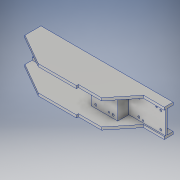
# Autodesk Inventor part: xtion_heatsink_mod
Saved by Autodesk Inventor 2017 (Build 210142000, 142)
## iProperties
Created: 2016-11-14
Part Number: xtion_heatsink_mod
Material: Aluminum 6061
Document SubType Name: Modeling
Designer: Alistair
Density: 2.7 g/cm^3
Appearance: Aluminum - Flat
Author: Alistair
Autodesk Inventor part; units mm, degrees
ref_plane "YZ Plane" through (0, 0, 0) normal (1, 0, 0) x (0, 1, 0)
ref_plane "XZ Plane" through (0, 0, 0) normal (0, 1, 0) x (-1, 0, 0)
ref_plane "XY Plane" through (0, 0, 0) normal (0, 0, 1) x (1, 0, 0)
sketch "Sketch1" plane through (0, 0, 0) normal (0, 0, 1) x (1, 0, 0)
  line L0 (-75, -10.5) -> (75, -10.5)
  line L1 (82, -9.5) -> (82, 9.5)
  line L2 (75, 10.5) -> (-75, 10.5)
  line L3 (-82, 9.5) -> (-82, -9.5)
  line L4 (-82, -10.5) -> (82, 10.5) construction
  line L5 (82, -10.5) -> (-82, 10.5) construction
  line L6 (75, 10.5) -> (82, 9.5)
  line L7 (0, 0) -> (27.9529, 0)
  line L8 (0, 0) -> (0, 6.9962)
  line L9 (-75, 10.5) -> (-82, 9.5)
  line L10 (75, -10.5) -> (82, -9.5)
  line L11 (-75, -10.5) -> (-82, -9.5)
  dimension "d0" = 21
  dimension "d1" = 164
  dimension "d4" = 7
  dimension "d5" = 1
  constraints: 24 end point, 6 symmetric about line, 5 point on line, 2 horizontal, 2 midpoint, 2 parallel, 1 perpendicular, 1 vertical
  measures "d0" distance of L5.end L4.start
  measures "d1" distance of L4.end L5.end
  measures "d4" distance from line of L1 L2.start
  measures "d5" vertical distance of L1.end L2.start
extrude "Extrusion1" add sketch "Sketch1" along normal blind 29
sketch "Sketch2" plane through (0, 0, 29) normal (0, 0, 1) x (1, 0, 0)
  line L0 (75, 10.5) -> (-75, 10.5) projected
  line L1 (-75, 10.5) -> (-82, 9.5) projected
  line L2 (-82, 9.5) -> (-82, -9.5) projected
  line L3 (-82, -9.5) -> (-75, -10.5) projected
  line L4 (-75, -10.5) -> (75, -10.5) projected
  line L5 (75, -10.5) -> (82, -9.5) projected
  line L6 (82, -9.5) -> (82, 9.5) projected
  line L7 (82, 9.5) -> (75, 10.5) projected
  line L8 (-74.8579, 8.5) -> (74.8579, 8.5)
  line L9 (74.8579, 8.5) -> (82, 7.4797)
  line L10 (82, -7.4797) -> (74.8579, -8.5)
  line L11 (74.8579, -8.5) -> (-74.8579, -8.5)
  line L12 (-74.8579, -8.5) -> (-82, -7.4797)
  line L13 (-82, 7.4797) -> (-74.8579, 8.5)
  point P0 (0, 0)
  dimension "d6" = 2
  constraints: 12 end point, 4 point on line
  measures "d6" distance between parallel lines of L0 L8
extrude "Extrusion2" cut sketch "Sketch2" against normal blind 15 contours L6 L10 L11 L12 L2 L13 L8 L9
sketch "Sketch3" plane through (0, 0, 14) normal (0, 0, 1) x (1, 0, 0)
  line L0 (-82, 7.4797) -> (-74.8579, 8.5) projected
  line L1 (-74.8579, 8.5) -> (74.8579, 8.5) projected
  line L2 (-74.8579, -8.5) -> (-82, -7.4797) projected
  line L3 (74.8579, -8.5) -> (-74.8579, -8.5) projected
  line L4 (82, -7.4797) -> (74.8579, -8.5) projected
  line L5 (74.8579, 8.5) -> (82, 7.4797) projected
  arc A0 (-82, -4.5) -> (-82, 4.5) centre (-83.875, 0) ccw
  line L6 (0, 0) -> (-13.589, 0)
  line L7 (-82, -7.4797) -> (-82, -4.5)
  line L8 (-82, 4.5) -> (-82, 7.4797)
  line L9 (0, 0) -> (0, 3.5906)
  arc A1 (82, 4.5) -> (82, -4.5) centre (83.875, 0) ccw
  line L10 (82, 7.4797) -> (82, 4.5)
  line L11 (82, -4.5) -> (82, -7.4797)
  arc A2 (-80.5, -5.4083) -> (-80.5, 5.4083) centre (-83.875, 0) ccw
  line L12 (-80.5, -5.4083) -> (-80.5, -7.694)
  line L13 (80.5, -7.694) -> (80.5, -5.4083)
  arc A3 (80.5, 5.4083) -> (80.5, -5.4083) centre (83.875, 0) ccw
  line L14 (80.5, 5.4083) -> (80.5, 7.694)
  line L15 (-80.5, 7.694) -> (-80.5, 5.4083)
  line L16 (-74.8579, 8.5) -> (74.8579, 8.5) projected
  line L17 (74.8579, -8.5) -> (-74.8579, -8.5) projected
  line L18 (10.5, 8.5) -> (30.5, 8.5)
  line L19 (30.5, 8.5) -> (30.5, -8.5)
  line L20 (30.5, -8.5) -> (10.5, -8.5)
  line L21 (10.5, -8.5) -> (10.5, 8.5)
  line L22 (82, -4.5) -> (82, 4.5)
  line L23 (82, -9.5) -> (82, 9.5) projected
  line L24 (-82, 4.5) -> (-82, -4.5)
  dimension "d10" = 9
  dimension "d11" = 3
  dimension "d12" = 1.5
  dimension "d13" = 1.5
  dimension "d14" = 1.5
  dimension "d15" = 1.5
  dimension "d16" = 1.5
  dimension "d17" = 1.5
  dimension "d18" = 20
  dimension "d19" = 51.5
  constraints: 32 end point, 10 point on circle, 9 point on line, 4 centre point, 4 parallel, 3 symmetric about line, 3 vertical, 2 horizontal, 1 collinear, 1 perpendicular, 1 other
  measures "d10" distance of L7.end L8.start
  measures "d11" distance edge to line of A0 L7
  measures "d12" radial gap between concentric circles of A0 A2
  measures "d13" radial gap between concentric circles of A1 A3
  measures "d14" distance between parallel lines of L10 L14
  measures "d15" distance between parallel lines of L11 L13
  measures "d16" distance between parallel lines of L8 L15
  measures "d17" distance between parallel lines of L7 L12
  measures "d18" distance between parallel lines of L19 L21
  measures "d19" distance between parallel lines of L11 L19
extrude "Extrusion3" cut sketch "Sketch3" against normal blind 7.5 contours L0 L1 L21 L3 L2 L12 A2 L15 | L1 L5 L14 A3 L13 L4 L3 L19 | L22 A1
sketch "Sketch4" plane through (0, 0, 6.5) normal (0, 0, 1) x (1, 0, 0)
  line L0 (-82, -4.5) -> (-82, 4.5) projected
  arc A0 (-82, -4.5) -> (-82, 4.5) centre (-83.875, 0) ccw projected
  line L1 (82, 4.5) -> (82, -4.5) projected
  arc A1 (82, 4.5) -> (82, -4.5) centre (83.875, 0) ccw projected
  line L2 (30.5, -8.5) -> (30.5, 8.5) projected
  line L3 (74.8579, -8.5) -> (30.5, -8.5) projected
  line L4 (80.5, -7.694) -> (74.8579, -8.5) projected
  line L5 (80.5, -5.4083) -> (80.5, -7.694) projected
  arc A2 (80.5, 5.4083) -> (80.5, -5.4083) centre (83.875, 0) ccw projected
  line L6 (80.5, 7.694) -> (80.5, 5.4083) projected
  line L7 (74.8579, 8.5) -> (80.5, 7.694) projected
  line L8 (30.5, 8.5) -> (74.8579, 8.5) projected
  line L9 (10.5, -8.5) -> (10.5, 8.5) projected
  line L10 (-74.8579, 8.5) -> (10.5, 8.5) projected
  line L11 (-80.5, 7.694) -> (-74.8579, 8.5) projected
  line L12 (-80.5, 5.4083) -> (-80.5, 7.694) projected
  arc A3 (-80.5, -5.4083) -> (-80.5, 5.4083) centre (-83.875, 0) ccw projected
  line L13 (-80.5, -7.694) -> (-80.5, -5.4083) projected
  line L14 (-74.8579, -8.5) -> (-80.5, -7.694) projected
  line L15 (10.5, -8.5) -> (-74.8579, -8.5) projected
  line L16 (4, 8.5) -> (4, -8.5)
  line L17 (-74.8579, 8.5) -> (74.8579, 8.5) projected
  line L18 (74.5, 8.5) -> (74.5, -8.5)
  line L19 (74.8579, -8.5) -> (-74.8579, -8.5) projected
  line L20 (63.5, 8.5) -> (63.5, -8.5)
  line L21 (-58, 6.5) -> (-35.889, 6.5)
  line L22 (-35.889, 6.5) -> (-35.889, -6.5)
  line L23 (-35.889, -6.5) -> (-58, -6.5)
  line L24 (-58, -6.5) -> (-58, 6.5)
  point P0 (0, 0)
  dimension "d22" = 6.5
  dimension "d23" = 7.5
  dimension "d24" = 11
  dimension "d25" = 24
  dimension "d26" = 2
  dimension "d27" = 2
  dimension "d28" = 22.111
  constraints: 14 end point, 6 point on line, 4 perpendicular, 2 parallel, 1 horizontal
  measures "d22" distance between parallel lines of L9 L16
  measures "d23" distance between parallel lines of L1 L18
  measures "d24" distance between parallel lines of L18 L20
  measures "d25" distance between parallel lines of L24 L0
  measures "d26" distance between parallel lines of L17 L21
  measures "d27" distance between parallel lines of L15 L23
  measures "d28" distance between parallel lines of L24 L22
extrude "Extrusion4" cut sketch "Sketch4" against normal through all contours L0 A0 | L1 A1 | L20 L8 L18 L3 | L15 L16 L10 L9 | L21 L22 L23 L24
sketch "Sketch5" plane through (0, 0, 0) normal (0, 0, -1) x (-1, 0, 0)
  line L0 (-4, -8.5) -> (-4, 8.5) projected
  line L1 (74.8579, 8.5) -> (-4, 8.5) projected
  line L2 (80.5, 7.694) -> (74.8579, 8.5) projected
  line L3 (80.5, 5.4083) -> (80.5, 7.694) projected
  arc A0 (80.5, 5.4083) -> (80.5, -5.4083) centre (83.875, 0) ccw projected
  line L4 (80.5, -7.694) -> (80.5, -5.4083) projected
  line L5 (74.8579, -8.5) -> (80.5, -7.694) projected
  line L6 (-4, -8.5) -> (74.8579, -8.5) projected
  line L7 (58, -6.5) -> (58, 6.5) projected
  line L8 (58, 6.5) -> (35.889, 6.5) projected
  line L9 (35.889, 6.5) -> (35.889, -6.5) projected
  line L10 (35.889, -6.5) -> (58, -6.5) projected
  line L11 (-63.5, -8.5) -> (-63.5, 8.5) projected
  line L12 (-30.5, 8.5) -> (-63.5, 8.5) projected
  line L13 (-30.5, -8.5) -> (-30.5, 8.5) projected
  line L14 (-63.5, -8.5) -> (-30.5, -8.5) projected
  line L15 (-10.5, 8.5) -> (-10.5, -8.5) projected
  line L16 (-30.5, -8.5) -> (-10.5, -8.5) projected
  line L17 (-30.5, -8.5) -> (-30.5, 8.5) projected
  line L18 (-10.5, 8.5) -> (-30.5, 8.5) projected
  line L19 (-74.5, 8.5) -> (-74.5, -8.5) projected
  line L20 (-74.8579, -8.5) -> (-74.5, -8.5) projected
  line L21 (-80.5, -7.694) -> (-74.8579, -8.5) projected
  line L22 (-80.5, -5.4083) -> (-80.5, -7.694) projected
  arc A1 (-80.5, -5.4083) -> (-80.5, 5.4083) centre (-83.875, 0) ccw projected
  line L23 (-80.5, 7.694) -> (-80.5, 5.4083) projected
  line L24 (-74.8579, 8.5) -> (-80.5, 7.694) projected
  line L25 (-74.5, 8.5) -> (-74.8579, 8.5) projected
  arc A2 (82, 4.5) -> (82, -4.5) centre (83.875, 0) ccw projected
  arc A3 (-82, -4.5) -> (-82, 4.5) centre (-83.875, 0) ccw projected
  line L26 (80.5, -5.4083) -> (80.5, -3.5178)
  line L27 (80.5, 5.4083) -> (80.5, 3.5178)
  line L28 (-80.5, 5.4083) -> (-80.5, 3.5178)
  line L29 (-80.5, -5.4083) -> (-80.5, -3.5178)
  point P0 (0, 0)
  constraints: 8 end point, 4 point on circle, 2 point on line, 1 parallel, 1 vertical
extrude "Extrusion5" cut sketch "Sketch5" against normal blind 4.5
sketch "Sketch6" plane through (0, 0, 14) normal (0, 0, 1) x (1, 0, 0)
  line L0 (10.5, 8.5) -> (10.5, -8.5) projected
  line L1 (30.5, -8.5) -> (10.5, -8.5) projected
  line L2 (30.5, -8.5) -> (30.5, 8.5) projected
  line L3 (10.5, 8.5) -> (30.5, 8.5) projected
  line L4 (14, 6.25) -> (14, -6.25) construction
  line L5 (27, 6.25) -> (27, -6.25) construction
  line L6 (10.5, 6.25) -> (30.5, 6.25) construction
  line L7 (30.5, -6.25) -> (10.5, -6.25) construction
  line L8 (0, 0) -> (2.4576, 0)
  point P0 (14, 0)
  dimension "d33" = 3.5
  dimension "d36" = 12.5
  dimension "d37" = 13
  constraints: 10 end point, 9 point on line, 4 perpendicular, 1 horizontal, 1 midpoint
  measures "d33" distance between parallel lines of L4 L0
  measures "d36" distance between parallel lines of L7 L6
  measures "d37" distance between parallel lines of L5 L4
hole "Hole1" at (14, 6.25, 14) at (14, -6.25, 14) at (27, -6.25, 14) at (27, 6.25, 14) direction (0, 0, -1) diameter 1.6 end through all
sketch "Sketch7" plane through (0, 0, 6.5) normal (0, 0, 1) x (1, 0, 0)
  line L0 (4, -8.5) -> (4, 8.5) projected
  line L1 (-74.8579, 8.5) -> (4, 8.5) projected
  line L2 (-80.5, 7.694) -> (-74.8579, 8.5) projected
  line L3 (-80.5, 5.4083) -> (-80.5, 7.694) projected
  arc A0 (-80.5, -5.4083) -> (-80.5, 5.4083) centre (-83.875, 0) ccw projected
  line L4 (-80.5, -7.694) -> (-80.5, -5.4083) projected
  line L5 (-74.8579, -8.5) -> (-80.5, -7.694) projected
  line L6 (4, -8.5) -> (-74.8579, -8.5) projected
  line L7 (-58, -6.5) -> (-58, 6.5) projected
  line L8 (-58, 6.5) -> (-35.889, 6.5) projected
  line L9 (-35.889, 6.5) -> (-35.889, -6.5) projected
  line L10 (-35.889, -6.5) -> (-58, -6.5) projected
  line L11 (-29.889, 5) -> (-20.889, 5)
  line L12 (-20.889, 5) -> (-20.889, -5)
  line L13 (-20.889, -5) -> (-29.889, -5)
  line L14 (-35.889, 3.25) -> (-29.889, 3.25)
  line L15 (-29.889, 1.75) -> (-35.889, 1.75)
  line L16 (-35.889, 1.75) -> (-35.889, 3.25)
  line L17 (-29.889, -1.75) -> (-35.889, -1.75)
  line L18 (-35.889, -1.75) -> (-35.889, -3.25)
  line L19 (-35.889, -3.25) -> (-29.889, -3.25)
  line L20 (0, 0) -> (-8.5394, 0)
  line L21 (-29.889, -5) -> (-29.889, -3.25)
  line L22 (-29.889, -1.75) -> (-29.889, 1.75)
  line L23 (-29.889, 3.25) -> (-29.889, 5)
  point P0 (-20.889, 0)
  point P1 (-29.889, 0)
  dimension "d46" = 1.5
  dimension "d47" = 1.5
  dimension "d48" = 3.5
  dimension "d50" = 10
  dimension "d51" = 9
  dimension "d52" = 6
  constraints: 26 end point, 6 parallel, 4 horizontal, 4 point on line, 2 collinear, 2 midpoint, 2 perpendicular
  measures "d46" distance between parallel lines of L15 L14
  measures "d47" distance between parallel lines of L19 L17
  measures "d48" distance between parallel lines of L15 L17
  measures "d50" distance between parallel lines of L13 L11
  measures "d51" distance between parallel lines of L12 L22
  measures "d52" distance of L14.start L14.end
extrude "Extrusion6" cut sketch "Sketch7" against normal blind 1.4 contours L9 L17 L22 L15 L14 L23 L11 L12 L13 L21 L19
sketch "Sketch8" plane through (0, 0, 6.5) normal (0, 0, 1) x (1, 0, 0)
  circle A0 centre (-34.139, 0) radius 1.75
  line L0 (-29.889, 1.75) -> (-35.889, 1.75) projected
  line L1 (0, 0) -> (-5.8224, 0)
  line L2 (-35.889, 1.75) -> (-35.889, -1.75) projected
  circle A1 centre (-17.639, 0) radius 1.75
  dimension "d55" = 3.5
  dimension "d56" = 3.5
  dimension "d57" = 16.5
  constraints: 2 centre point, 2 end point, 2 tangent, 1 horizontal, 1 point on line
  measures "d55" diameter of A0
  measures "d56" diameter of A1
  measures "d57" distance of A0.centre A1.centre
extrude "Extrusion7" add sketch "Sketch8" along normal blind 1.58 contours A0 | A1
sketch "Sketch9" plane through (0, 0, 4.5) normal (0, 0, -1) x (-1, 0, 0)
  line L0 (29.889, 3.25) -> (29.889, 5) projected
  line L1 (35.889, 3.25) -> (29.889, 3.25) projected
  line L2 (35.889, 1.75) -> (35.889, 3.25) projected
  line L3 (35.889, -3.25) -> (35.889, -1.75) projected
  line L4 (29.889, -3.25) -> (35.889, -3.25) projected
  line L5 (29.889, -5) -> (29.889, -3.25) projected
  line L6 (20.889, -5) -> (29.889, -5) projected
  line L7 (20.889, 5) -> (20.889, -5) projected
  line L8 (29.889, 5) -> (20.889, 5) projected
  line L9 (35.889, 1.75) -> (35.889, -1.75)
  line L10 (19.389, 8.5) -> (19.389, -8.5)
  line L11 (19.389, -6.5) -> (31.389, -6.5)
  line L12 (31.389, -8.5) -> (31.389, -4.75)
  line L13 (31.389, -4.75) -> (35.889, -4.75)
  line L14 (35.889, 4.75) -> (31.389, 4.75)
  line L15 (31.389, 4.75) -> (31.389, 8.5)
  line L16 (31.389, 6.5) -> (19.389, 6.5)
  line L17 (35.889, 3.25) -> (35.889, 4.75)
  line L18 (35.889, 6.5) -> (35.889, -6.5) projected
  line L19 (35.889, -3.25) -> (35.889, -4.75)
  line L20 (58, 6.5) -> (35.889, 6.5) projected
  line L21 (58, -6.5) -> (58, 6.5) projected
  line L22 (35.889, -6.5) -> (58, -6.5) projected
  line L23 (35.889, 6.5) -> (35.889, -6.5) projected
  line L24 (80.5, -3.5178) -> (80.5, -7.694) projected
  arc A0 (80.5, 3.5178) -> (80.5, -3.5178) centre (83.875, 0) ccw projected
  line L25 (80.5, 7.694) -> (80.5, 3.5178) projected
  line L26 (74.8579, 8.5) -> (80.5, 7.694) projected
  line L27 (-4, 8.5) -> (74.8579, 8.5) projected
  line L28 (-4, -8.5) -> (-4, 8.5) projected
  line L29 (74.8579, -8.5) -> (-4, -8.5) projected
  line L30 (80.5, -7.694) -> (74.8579, -8.5) projected
  point P0 (0, 0)
  dimension "d60" = 1.5
  constraints: 20 end point, 10 point on line, 1 vertical
  measures "d60" distance between parallel lines of L8 L16
extrude "Extrusion8" add sketch "Sketch9" along normal blind 1.5 contours L1 L2 L9 L3 L4 L5 L6 L7 L8 L0 | L0 L8 L7 L6 L5 L4 L18 L13 L12 L11 L10 L16 L15 L14 L17 L1 | L16 L10 L27 L15 | L11 L12 L29 L10
chamfer "Chamfer1" distance 1.5 angle 45 3 edges at (-19.389, 0, 3) (-31.389, 6.625, 3) (-31.389, -6.625, 3)
sketch "Sketch10" plane through (-34.139, 0, 8.08) normal (0, 0, 1) x (1, 0, 0)
  circle A0 centre (0, 0) radius 1.75 projected
  circle A1 centre (16.5, 0) radius 1.75 projected
  point P0 (34.139, 0)
hole "Hole2" at (-34.139, 0, 8.08) at (-17.639, 0, 8.08) direction (0, 0, -1) diameter 1.6 end through all
sketch "Sketch11" plane through (0, 0, 6.5) normal (0, 0, 1) x (1, 0, 0)
  line L0 (63.5, -8.5) -> (63.5, 8.5) projected
  line L1 (30.5, 8.5) -> (63.5, 8.5) projected
  line L2 (30.5, -8.5) -> (30.5, 8.5) projected
  line L3 (63.5, -8.5) -> (30.5, -8.5) projected
  line L4 (74.8579, 8.5) -> (-74.8579, 8.5) projected
  line L5 (59, 8.5) -> (59, -8.5)
  point P0 (0, 0)
  dimension "d73" = 4.5
  constraints: 2 end point, 2 point on line, 1 perpendicular
  measures "d73" distance between parallel lines of L0 L5
extrude "Extrusion9" cut sketch "Sketch11" against normal blind 0.8 contours L3 L2 L1 L5
sketch "Sketch12" plane through (0, 0, 5.7) normal (0, 0, 1) x (1, 0, 0)
  line L0 (30.5, -8.5) -> (30.5, 8.5) projected
  line L1 (59, -8.5) -> (30.5, -8.5) projected
  line L2 (59, 8.5) -> (59, -8.5) projected
  line L3 (30.5, 8.5) -> (59, 8.5) projected
  line L4 (-74.8579, 8.5) -> (74.8579, 8.5) projected
  line L5 (38, 6.25) -> (38, -6.25) construction
  line L6 (74.8579, -8.5) -> (-74.8579, -8.5) projected
  line L7 (54.5, 6.25) -> (54.5, -6.25) construction
  line L8 (38, 6.25) -> (54.5, 6.25) construction
  line L9 (38, -6.25) -> (54.5, -6.25) construction
  line L10 (0, 0) -> (7.4065, 0)
  circle A0 centre (27, -6.25) radius 0.8 projected
  point P0 (38, 0)
  dimension "d77" = 16.5
  dimension "d78" = 12.5
  dimension "d86" = 11
  constraints: 10 end point, 4 coincident, 3 perpendicular, 1 horizontal, 1 midpoint, 1 point on line, 1 vertical
  measures "d77" distance between parallel lines of L7 L5
  measures "d78" distance between parallel lines of L8 L9
  measures "d86" distance of L5.end A0.centre
hole "Hole3" at (38, 6.25, 5.7) at (38, -6.25, 5.7) at (54.5, -6.25, 5.7) at (54.5, 6.25, 5.7) direction (0, 0, -1) diameter 1.6 end through all
sketch "Sketch13" plane through (-75, 10.5, 0) normal (0, 1, 0) x (1, 0, 0)
  line L0 (39.111, -4.5) -> (17, -4.5) projected
  line L1 (17, -6.5) -> (17, -4.5) projected
  line L2 (39.111, -6.5) -> (17, -6.5) projected
  line L3 (39.111, -6.5) -> (39.111, -4.5) projected
  line L4 (150, 0) -> (0, 0) projected
  line L5 (0, 0) -> (0, -29) projected
  line L6 (150, -29) -> (0, -29) projected
  line L7 (150, 0) -> (150, -29) projected
  line L8 (150, -29) -> (0, -29) projected
  line L9 (39.111, -29) -> (45.711, -29)
  line L10 (45.711, -29) -> (45.711, -22)
  line L11 (45.711, -22) -> (39.111, -22)
  line L12 (39.111, -22) -> (39.111, -29)
  point P0 (75, 0)
  dimension "d87" = 6.6
  dimension "d88" = 7
  constraints: 8 end point, 2 parallel, 1 collinear, 1 horizontal, 1 perpendicular, 1 point on line
  measures "d87" distance between parallel lines of L10 L12
  measures "d88" distance between parallel lines of L6 L11
extrude "Extrusion10" cut sketch "Sketch13" against normal up to next contours L6 L12 L11 L10
sketch "Sketch14" plane through (-75, -10.5, 0) normal (0, -1, 0) x (1, 0, 0)
  line L0 (0, 29) -> (150, 29) projected
  line L1 (0, 0) -> (0, 29) projected
  line L2 (0, 0) -> (150, 0) projected
  line L3 (150, 0) -> (150, 29) projected
  line L4 (0, 29) -> (150, 29) projected
  line L5 (28, 29) -> (135, 29)
  line L6 (135, 29) -> (135, 25.5)
  line L7 (135, 25.5) -> (28, 25.5)
  line L8 (28, 25.5) -> (28, 29)
  line L9 (-7, 0) -> (0, 0) projected
  line L10 (0, 0) -> (0, 29) projected
  line L11 (-7, 29) -> (0, 29) projected
  line L12 (-7, 0) -> (-7, 29) projected
  line L13 (135, 25.5) -> (86, 25.5)
  line L14 (86, 25.5) -> (86, 24)
  line L15 (86, 24) -> (135, 24)
  line L16 (135, 24) -> (135, 25.5)
  point P0 (75, 0)
  dimension "d91" = 107
  dimension "d92" = 35
  dimension "d93" = 3.5
  dimension "d94" = 5
  dimension "d95" = 49
  constraints: 16 end point, 4 parallel, 2 horizontal, 2 perpendicular, 1 point on line
  measures "d91" distance between parallel lines of L6 L8
  measures "d92" distance between parallel lines of L8 L12
  measures "d93" distance between parallel lines of L0 L7
  measures "d94" distance between parallel lines of L15 L0
  measures "d95" distance between parallel lines of L16 L14
extrude "Extrusion11" cut sketch "Sketch14" against normal through all contours L0 L6 L7 L8 | L16 L15 L14 L7
sketch "Sketch15" plane through (0, 0, 4.5) normal (0, 0, -1) x (-1, 0, 0)
  circle A0 centre (-51.2525, 6.9125) radius 0.5 projected
  circle A1 centre (-41.1992, -6.949) radius 0.5 projected
  point P0 (0, 0)
  constraints: 2 coincident
hole "Hole4" at (51.2525, 6.9125, 4.5) at (41.1992, -6.949, 4.5) direction (0, 0, 1) diameter 1.1 end through all
sketch "Sketch16" plane through (0, 0, 4.5) normal (0, 0, -1) x (-1, 0, 0)
  circle A0 centre (-51.2525, 6.9125) radius 0.55 projected
  circle A1 centre (-41.1992, -6.949) radius 0.55 projected
  circle A2 centre (-54.5, -6.25) radius 0.8 projected
  circle A3 centre (-38, 6.25) radius 0.8 projected
  circle A4 centre (-38, -6.25) radius 0.8 projected
  circle A5 centre (-54.5, 6.25) radius 0.8 projected
  circle A6 centre (-27, -6.25) radius 0.8 projected
  circle A7 centre (-14, 6.25) radius 0.8 projected
  circle A8 centre (-14, -6.25) radius 0.8 projected
  circle A9 centre (-27, 6.25) radius 0.8 projected
  line L0 (-10.5, 8.5) -> (-10.5, -8.5) projected
  line L1 (-63.5, 8.5) -> (-10.5, 8.5) projected
  line L2 (-63.5, -8.5) -> (-63.5, 8.5) projected
  line L3 (-10.5, -8.5) -> (-63.5, -8.5) projected
  line L4 (-63.5, 8.5) -> (-10.5, 8.5) projected
  line L5 (-28.1, 8.5) -> (-28.1, -8.5)
  line L6 (-10.5, -8.5) -> (-63.5, -8.5) projected
  line L7 (-12, 8.5) -> (-12, -8.5)
  point P0 (0, 0)
  dimension "d105" = 16.1
  dimension "d106" = 1.5
  constraints: 4 end point, 4 point on line, 2 perpendicular
  measures "d105" distance between parallel lines of L7 L5
  measures "d106" distance between parallel lines of L0 L7
extrude "Extrusion12" cut sketch "Sketch16" against normal blind 8 contours L7 L3 L5 L1
sketch "Sketch17" plane through (0, 0, 12.5) normal (0, 0, -1) x (-1, 0, 0)
  circle A0 centre (-24, -6) radius 0.5 projected
  circle A1 centre (-17, 6) radius 0.5 projected
  point P0 (0, 0)
  constraints: 2 coincident
hole "Hole5" at (24, -6, 12.5) at (17, 6, 12.5) direction (0, 0, 1) diameter 1.1 end through all
sketch "Sketch18" plane through (-75, 10.5, 0) normal (0, 1, 0) x (1, 0, 0)
  line L0 (130.3, -5.7) -> (128.7, -5.7) projected
  line L1 (132.9, 5.419) -> (132.9, -6.6)
  line L2 (39.111, -5.1) -> (39.111, -6.5) projected
  line L3 (39.111, -6.5) -> (39.111, -4.5) projected
  line L4 (39.111, -4.5) -> (39.111, -3) projected
  line L5 (39.111, -4.5) -> (39.111, -3) projected
  line L6 (39.111, -6.5) -> (39.111, -4.5) projected
  line L7 (39.111, -6.5) -> (39.111, -5.1) projected
  line L8 (39.111, -5.1) -> (39.111, -6.5) projected
  line L9 (39.111, -6.5) -> (39.111, -5.1) projected
  line L10 (33.911, 5.419) -> (132.9, 5.419)
  line L11 (39.111, -25.5) -> (28, -25.5) projected
  line L12 (57.361, -25.5) -> (102, -25.5)
  line L13 (132.9, -6.6) -> (119.5788, -6.6) construction
  line L14 (150, 0) -> (0, 0) construction
  line L15 (132.9, -6.6) -> (117.3207, -6.5805)
  line L16 (102.8, -12.5) -> (101.2, -12.5) projected
  line L17 (102.8, -14) -> (101.2, -14) projected
  line L18 (102, -25.5) -> (117.3207, -6.5805)
  line L19 (112.2, -4.5) -> (113.8, -4.5) projected
  line L20 (113.8, -5.7) -> (112.2, -5.7) projected
  line L21 (102, -14) -> (102, -16.4025) construction
  line L22 (33.911, -12) -> (57.361, -25.5)
  line L23 (45.711, -25.5) -> (86, -25.5) projected
  line L24 (56.561, -4.5) -> (58.161, -4.5) projected
  line L25 (58.161, -8.08) -> (56.561, -8.08) projected
  line L26 (57.361, -8.08) -> (57.361, -12) construction
  line L27 (33.911, 5.419) -> (33.911, -12)
  point P0 (75, 0)
  point P1 (39.111, -6.5)
  dimension "d116" = 2.6
  dimension "d118" = 6.6
  dimension "d119" = 129
  dimension "d120" = 12
  constraints: 20 end point, 4 vertical, 3 point on line, 2 midpoint, 2 perpendicular, 1 horizontal
  measures "d116" distance from line of L1 L0.start
  measures "d118" distance between parallel lines of L13 L14
  measures "d119" angle of L18 L12
  measures "d120" distance from line of L14 L22.start
extrude "Extrusion13" cut sketch "Sketch18" against normal through all keep common part
equation "\"d14\" = d13"
equation "\"d15\" = d13"
equation "\"d16\" = d12"
equation "\"d17\" = d12"
equation "\"d47\" = d46"
equation "\"d56\" = d55"
body "Solid1"
